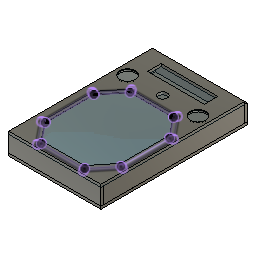
Enclosure Model v2 (Autodesk Fusion 360 design; units mm, degrees)
Autodesk Fusion 360 part; units mm, degrees
sketch "Sketch1" plane through (0, 0, 0) normal (0, 0, 1) x (1, 0, 0) in component "Back"
  line L0 (107.95, 171.45) -> (-107.95, 171.45)
  line L1 (-107.95, 171.45) -> (-107.95, -171.45)
  line L2 (-107.95, -171.45) -> (107.95, -171.45)
  line L3 (107.95, -171.45) -> (107.95, 171.45)
  line L4 (107.95, 171.45) -> (-107.95, -171.45) construction
  line L5 (-107.95, 171.45) -> (107.95, -171.45) construction
  dimension "d1" = 215.9
  dimension "d2" = 342.9
  constraint horizontal L0
  constraint perpendicular L0 L1
  constraint parallel L0 L2
  constraint parallel L1 L3
  constraint coincident L4 origin
  constraint coincident L5 origin
  measures "d1" distance of L1.end L2.end
  measures "d2" distance of L0.end L1.end
extrude "Extrude1" add sketch "Sketch1" along normal blind 6.35 makes body 1 in component "Back"
ref_plane "WorkPlane1" through (0, 131.445, 0) normal (0, 1, 0) x (0, 0, 1) in component "Top/Bottom"
sketch "Sketch1 (2)" plane through (0, 131.445, 0) normal (0, 1, 0) x (1, 0, 0) in component "Top/Bottom"
  line L0 (-101.6, 0) -> (102.87, 0)
  line L1 (102.87, 0) -> (102.87, -50.8)
  line L2 (102.87, -50.8) -> (-101.6, -50.8)
  line L3 (-101.6, -50.8) -> (-101.6, 0)
  dimension "d36" = 204.47
  dimension "d37" = 50.8
  constraint horizontal L0
  constraint vertical L1
  constraint horizontal L2
  constraint vertical L3
  measures "d36" distance of L0.start L0.end
  measures "d37" distance of L0.start L2.end
sketch "Sketch4" plane through (0, 0, 6.35) normal (0, 0, 1) x (-1, 0, 0) in component "Top/Bottom"
  line L0 (-107.95, 171.45) -> (-107.95, -171.45)
  line L1 (-107.95, -171.45) -> (107.95, -171.45)
  line L2 (107.95, -171.45) -> (107.95, 171.45)
  line L3 (107.95, 171.45) -> (-107.95, 171.45)
  line L4 (107.95, -171.45) -> (-107.95, -171.45)
  line L5 (-107.95, -171.45) -> (-107.95, -165.1)
  line L6 (-107.95, -165.1) -> (107.95, -165.1)
  line L7 (107.95, -165.1) -> (107.95, -171.45)
  dimension "d43" = 215.9
  dimension "d44" = 6.35
  constraint horizontal L4
  constraint vertical L5
  constraint horizontal L6
  constraint vertical L7
  constraint coincident L1.end L2.start
  measures "d43" distance of L1.end L0.end
  measures "d44" distance of L1.end L6.end
extrude "Extrude2" add sketch "Sketch4" along normal blind 38.1 separate body contours L0 L1 L2 L4 L5 L6 L7 makes body 2 in component "Top/Bottom"
mirror "Mirror1" about plane through (0, 0, 0) normal (0, 1, 0) of bodies 2 makes body 3 in component "Top/Bottom"
sketch "Sketch1 (3)" plane through (0, 0, 6.35) normal (0, 0, 1) x (-1, 0, 0) in component "Left"
  line L0 (-107.95, 171.45) -> (-107.95, -171.45)
  line L1 (-107.95, -171.45) -> (107.95, -171.45)
  line L2 (107.95, -171.45) -> (107.95, 171.45)
  line L3 (107.95, 171.45) -> (-107.95, 171.45)
  line L4 (107.95, -171.45) -> (107.95, -165.1) construction
  line L5 (107.95, -165.1) -> (101.6, -165.1)
  line L6 (101.6, -165.1) -> (101.6, 165.1)
  line L7 (101.6, 165.1) -> (107.95, 165.1)
  line L8 (107.95, 165.1) -> (107.95, -165.1)
  dimension "d49" = 6.35
  dimension "d50" = 330.2
  constraint coincident L1.end L2.start
  constraint coincident L2 L4.end
  constraint perpendicular L1 L4
  constraint horizontal L5
  constraint vertical L6
  constraint horizontal L7
  constraint vertical L8
  measures "d49" distance of L4.end L5.end
  measures "d50" distance of L4.end L7.end
extrude "Extrude1'" add sketch "Sketch1 (3)" along normal blind 38.1 separate body contours L2 L5 L6 L7 L8 makes body 4 in component "Left"
mirror "Mirror1'" about plane through (0, 0, 0) normal (1, 0, 0) of bodies 4 makes body 5 in component "Left"
sketch "Sketch1 (4)" plane through (0, 0, 44.45) normal (0, 0, 1) x (-1, 0, 0) in component "Lid"
  line L0 (107.95, -165.1) -> (-107.95, -165.1)
  line L1 (-107.95, -165.1) -> (-107.95, -171.45)
  line L2 (-107.95, -171.45) -> (107.95, -171.45)
  line L3 (107.95, -171.45) -> (107.95, -165.1)
  line L4 (107.95, -171.45) -> (-107.95, -171.45)
  line L5 (-107.95, -171.45) -> (-107.95, 171.45)
  line L6 (-107.95, 171.45) -> (107.95, 171.45)
  line L7 (107.95, 171.45) -> (107.95, -171.45)
  dimension "d55" = 215.9
  dimension "d56" = 342.9
  constraint horizontal L4
  constraint vertical L5
  constraint horizontal L6
  constraint vertical L7
  constraint coincident L2.end L3.start
  measures "d55" distance of L2.end L1.end
  measures "d56" distance of L2.end L6.end
extrude "Extrude1''" add sketch "Sketch1 (4)" along normal blind 6.35 separate body contours L0 L5 L6 L7 makes body 6 in component "Lid"
sketch "Sketch2" plane through (0, 0, 50.8) normal (0, 0, 1) x (-1, 0, 0) in component "Lid"
  line L0 (107.95, 171.45) -> (-107.95, 171.45)
  line L1 (-107.95, 171.45) -> (-107.95, -165.1)
  line L2 (-107.95, -165.1) -> (107.95, -165.1)
  line L3 (107.95, -165.1) -> (107.95, 171.45)
  line L4 (0, 171.45) -> (0, 152.4) construction
  line L5 (0, 152.4) -> (0, -50.8) construction
  line L6 (0, -50.8) -> (0, 50.8) construction
  line L7 (0, 50.8) -> (57.15, 50.8) construction
  line L8 (0, 152.4) -> (50.8, 152.4)
  line L9 (50.8, 152.4) -> (50.8, 105.41) construction
  line L10 (50.8, 105.41) -> (88.9, 105.41) construction
  line L11 (50.8, 152.4) -> (88.9, 105.41)
  line L12 (88.9, 105.41) -> (88.9, -8.89)
  line L13 (88.9, -8.89) -> (50.8, -8.89) construction
  line L14 (50.8, -8.89) -> (50.8, -55.88) construction
  line L15 (88.9, -8.89) -> (50.8, -55.88)
  line L16 (50.8, -55.88) -> (0, -55.88)
  line L17 (0, -55.88) -> (0, 152.4)
  dimension "d59" = 19.05
  dimension "d60" = 203.2
  dimension "d61" = 101.6
  dimension "d62" = 57.15
  dimension "d63" = 50.8
  dimension "d64" = 46.99
  dimension "d65" = 38.1
  dimension "d66" = 114.3
  dimension "d67" = 38.1
  dimension "d68" = 46.99
  dimension "d69" = 50.8
  constraint midpoint L0 L4.start
  constraint perpendicular L0 L4
  constraint parallel L4 L5
  constraint parallel L5 L6
  constraint perpendicular L6 L7
  constraint perpendicular L4 L8
  constraint perpendicular L8 L9
  constraint perpendicular L9 L10
  constraint perpendicular L10 L12
  constraint perpendicular L12 L13
  constraint perpendicular L13 L14
  constraint perpendicular L14 L16
  measures "d59" distance of L4.start L4.end
  measures "d60" distance of L4.end L5.end
  measures "d61" distance of L5.end L6.end
  measures "d62" distance of L6.end L7.end
  measures "d63" distance of L4.end L8.end
  measures "d64" distance of L8.end L9.end
  measures "d65" distance of L9.end L10.end
  measures "d66" distance of L10.end L12.end
  measures "d67" distance of L12.end L13.end
  measures "d68" distance of L13.end L14.end
  measures "d69" distance of L14.end L16.end
extrude "Extrude2'" cut sketch "Sketch2" against normal up to surface (6.35 mm away) contours L8 L11 L12 L15 L16 L17 bodies 6 in component "Lid"
mirror "Mirror1''" about plane through (0, 0, 0) normal (1, 0, 0) of "Extrude2'" in component "Lid"
sketch "Sketch3" plane through (0, 0, 50.8) normal (0, 0, 1) x (-1, 0, 0) in component "Lid"
  line L0 (107.95, 171.45) -> (-107.95, 171.45)
  line L1 (-107.95, 171.45) -> (-107.95, -165.1)
  line L2 (-107.95, -165.1) -> (107.95, -165.1)
  line L3 (107.95, -165.1) -> (107.95, 171.45)
  line L4 (50.8, -55.88) -> (-50.8, -55.88)
  line L5 (-50.8, -55.88) -> (-88.9, -8.89)
  line L6 (-88.9, -8.89) -> (-88.9, 105.41)
  line L7 (-88.9, 105.41) -> (-50.8, 152.4)
  line L8 (-50.8, 152.4) -> (50.8, 152.4)
  line L9 (50.8, 152.4) -> (88.9, 105.41)
  line L10 (88.9, 105.41) -> (88.9, -8.89)
  line L11 (88.9, -8.89) -> (50.8, -55.88)
  circle A0 centre (0, -81.28) radius 10.668
  dimension "d74" = 21.336
  dimension "d75" = 25.4
  measures "d74" diameter of A0
  measures "d75" distance of L4 A0.centre
extrude "Extrude3" cut sketch "Sketch3" against normal up to surface (6.35 mm away) contours A0 bodies 6 in component "Lid"
sketch "Sketch4 (2)" plane through (0, 0, 50.8) normal (0, 0, 1) x (-1, 0, 0) in component "Lid"
  circle A0 centre (0, -81.28) radius 10.668
  line L0 (107.95, 171.45) -> (-107.95, 171.45)
  line L1 (-107.95, 171.45) -> (-107.95, -165.1)
  line L2 (-107.95, -165.1) -> (107.95, -165.1)
  line L3 (107.95, -165.1) -> (107.95, 171.45)
  line L4 (50.8, -55.88) -> (-50.8, -55.88)
  line L5 (-50.8, -55.88) -> (-88.9, -8.89)
  line L6 (-88.9, -8.89) -> (-88.9, 105.41)
  line L7 (-88.9, 105.41) -> (-50.8, 152.4)
  line L8 (-50.8, 152.4) -> (50.8, 152.4)
  line L9 (50.8, 152.4) -> (88.9, 105.41)
  line L10 (88.9, 105.41) -> (88.9, -8.89)
  line L11 (88.9, -8.89) -> (50.8, -55.88)
  line L12 (66.675, -144.018) -> (-66.675, -144.018)
  line L13 (-66.675, -144.018) -> (-66.675, -112.268)
  line L14 (-66.675, -112.268) -> (66.675, -112.268)
  line L15 (66.675, -112.268) -> (66.675, -144.018)
  line L16 (66.675, -144.018) -> (-66.675, -112.268) construction
  line L17 (-66.675, -144.018) -> (66.675, -112.268) construction
  point P0 (0, -128.143)
  dimension "d78" = 133.35
  dimension "d79" = 31.75
  dimension "d80" = 30.988
  constraint horizontal L12
  constraint perpendicular L12 L13
  constraint parallel L12 L14
  constraint parallel L13 L15
  constraint coincident L16 P0
  constraint coincident L17 P0
  measures "d78" distance of L13.end L14.end
  measures "d79" distance of L12.end L13.end
  measures "d80" distance of A0.centre L14
extrude "Extrude4" cut sketch "Sketch4 (2)" against normal up to surface (6.35 mm away) contours L12 L13 L14 L15 bodies 6 in component "Lid"
sketch "Sketch5" plane through (0, 0, 44.45) normal (0, 0, -1) x (1, 0, 0) in component "Lid"
  line L0 (-66.675, -144.018) -> (-66.675, -112.268)
  line L1 (-66.675, -112.268) -> (66.675, -112.268)
  line L2 (66.675, -112.268) -> (66.675, -144.018)
  line L3 (66.675, -144.018) -> (-66.675, -144.018)
  circle A0 centre (0, -81.28) radius 10.668
  line L4 (50.8, -55.88) -> (-50.8, -55.88)
  line L5 (-50.8, -55.88) -> (-88.9, -8.89)
  line L6 (-88.9, -8.89) -> (-88.9, 105.41)
  line L7 (-88.9, 105.41) -> (-50.8, 152.4)
  line L8 (-50.8, 152.4) -> (50.8, 152.4)
  line L9 (50.8, 152.4) -> (88.9, 105.41)
  line L10 (88.9, 105.41) -> (88.9, -8.89)
  line L11 (88.9, -8.89) -> (50.8, -55.88)
  line L12 (107.95, 171.45) -> (-107.95, 171.45)
  line L13 (-107.95, 171.45) -> (-107.95, -165.1)
  line L14 (-107.95, -165.1) -> (107.95, -165.1)
  line L15 (107.95, -165.1) -> (107.95, 171.45)
  line L16 (-88.9, -8.89) -> (-50.8, -55.88)
  line L17 (-50.8, -55.88) -> (50.8, -55.88)
  line L18 (-88.9, 105.41) -> (-88.9, -8.89)
  line L19 (50.8, -55.88) -> (88.9, -8.89)
  line L20 (88.9, -8.89) -> (88.9, 105.41)
  line L21 (88.9, 105.41) -> (50.8, 152.4)
  line L22 (-50.8, 152.4) -> (-88.9, 105.41)
  line L23 (50.8, 152.4) -> (-50.8, 152.4)
  line L24 (-50.8, -55.88) -> (50.8, -55.88)
  line L25 (50.8, -55.88) -> (88.9, -8.89)
  line L26 (88.9, 105.41) -> (50.8, 152.4)
  line L27 (50.8, 152.4) -> (-50.8, 152.4)
  line L28 (-50.8, 152.4) -> (-88.9, 105.41)
  line L29 (-88.9, 105.41) -> (-88.9, -8.89)
  line L30 (-88.9, -8.89) -> (-50.8, -55.88)
  constraint coincident L4.end L5.start
  constraint coincident L4.start L11.end
  constraint coincident L10.end L11.start
  constraint coincident L9.end L10.start
  constraint coincident L8.end L9.start
  constraint coincident L7.end L8.start
  constraint coincident L6.end L7.start
  constraint coincident L5.end L6.start
sketch "Sketch1 (5)" plane through (0, 0, 44.45) normal (0, 0, -1) x (1, 0, 0) in component "Punch Box"
  line L0 (-50.8, 152.4) -> (50.8, 152.4)
  line L1 (-88.9, 105.41) -> (-50.8, 152.4)
  line L2 (-88.9, -8.89) -> (-88.9, 105.41)
  line L3 (-50.8, -55.88) -> (-88.9, -8.89)
  line L4 (50.8, -55.88) -> (-50.8, -55.88)
  line L5 (88.9, -8.89) -> (50.8, -55.88)
  line L6 (88.9, 105.41) -> (88.9, -8.89)
  line L7 (50.8, 152.4) -> (88.9, 105.41)
  line L8 (53.8264, 158.75) -> (95.25, 107.6609)
  line L9 (95.25, 107.6609) -> (95.25, -11.1409)
  line L10 (95.25, -11.1409) -> (53.8264, -62.23)
  line L11 (53.8264, -62.23) -> (-53.8264, -62.23)
  line L12 (-53.8264, -62.23) -> (-95.25, -11.1409)
  line L13 (-95.25, -11.1409) -> (-95.25, 107.6609)
  line L14 (-95.25, 107.6609) -> (-53.8264, 158.75)
  line L15 (-53.8264, 158.75) -> (53.8264, 158.75)
  line L16 (98.425, 108.7863) -> (98.425, -12.2663)
  line L17 (98.425, -12.2663) -> (55.3396, -65.405)
  line L18 (55.3396, -65.405) -> (-55.3396, -65.405)
  line L19 (-55.3396, -65.405) -> (-98.425, -12.2663)
  line L20 (-98.425, -12.2663) -> (-98.425, 108.7863)
  line L21 (-98.425, 108.7863) -> (-55.3396, 161.925)
  line L22 (-55.3396, 161.925) -> (55.3396, 161.925)
  line L23 (55.3396, 161.925) -> (98.425, 108.7863)
  dimension "d83" = -6.35
  dimension "d84" = -9.525
extrude "Extrude1'''" add sketch "Sketch1 (5)" along normal blind 34.925 separate body contours L16 L17 L18 L19 L20 L21 L22 L23 makes body 7 in component "Punch Box"
sketch "Sketch5 (2)" plane through (0, 0, 9.525) normal (0, 0, -1) x (1, 0, 0) in component "Punch Box"
  line L0 (-95.25, 107.6609) -> (-53.8264, 158.75)
  line L1 (-53.8264, 158.75) -> (53.8264, 158.75)
  line L2 (53.8264, 158.75) -> (95.25, 107.6609)
  line L3 (95.25, 107.6609) -> (95.25, -11.1409)
  line L4 (95.25, -11.1409) -> (53.8264, -62.23)
  line L5 (53.8264, -62.23) -> (-53.8264, -62.23)
  line L6 (-53.8264, -62.23) -> (-95.25, -11.1409)
  line L7 (-95.25, -11.1409) -> (-95.25, 107.6609)
  line L8 (55.3396, 161.925) -> (-55.3396, 161.925)
  line L9 (-55.3396, 161.925) -> (-98.425, 108.7863)
  line L10 (-98.425, 108.7863) -> (-98.425, -12.2663)
  line L11 (-98.425, -12.2663) -> (-55.3396, -65.405)
  line L12 (-55.3396, -65.405) -> (55.3396, -65.405)
  line L13 (55.3396, -65.405) -> (98.425, -12.2663)
  line L14 (98.425, -12.2663) -> (98.425, 108.7863)
  line L15 (98.425, 108.7863) -> (55.3396, 161.925)
  line L16 (55.3396, -65.405) -> (-55.3396, -65.405)
  line L17 (-55.3396, -65.405) -> (-98.425, -12.2663)
  line L18 (-98.425, 108.7863) -> (-98.425, -12.2663)
  line L19 (-98.425, 108.7863) -> (-55.3396, 161.925)
  line L20 (-55.3396, 161.925) -> (55.3396, 161.925)
  line L21 (98.425, 108.7863) -> (55.3396, 161.925)
  line L22 (98.425, 108.7863) -> (98.425, -12.2663)
  line L23 (98.425, -12.2663) -> (55.3396, -65.405)
  constraint coincident L12.end L13.start
  constraint coincident L11.end L12.start
  constraint coincident L10.end L11.start
  constraint coincident L9.end L10.start
  constraint coincident L8.end L9.start
  constraint coincident L8.start L15.end
  constraint coincident L14.end L15.start
  constraint parallel L15 L21
  constraint coincident L13.end L14.start
extrude "Extrude2''" add sketch "Sketch5 (2)" along normal blind 3.175 separate body contours L0 L1 L2 L3 L4 L5 L6 L7 makes body 8 in component "Punch Box"
sketch "Sketch1 (6)" plane through (0, 0, 44.45) normal (0, 0, -1) x (1, 0, 0) in component "Punch Pad"
  line L0 (53.8264, -62.23) -> (-53.8264, -62.23)
  line L1 (-53.8264, -62.23) -> (-95.25, -11.1409)
  line L2 (-95.25, -11.1409) -> (-95.25, 107.6609)
  line L3 (95.25, -11.1409) -> (53.8264, -62.23)
  line L4 (95.25, 107.6609) -> (95.25, -11.1409)
  line L5 (53.8264, 158.75) -> (95.25, 107.6609)
  line L6 (-53.8264, 158.75) -> (53.8264, 158.75)
  line L7 (-95.25, 107.6609) -> (-53.8264, 158.75)
extrude "Extrude1''''" add sketch "Sketch1 (5)" along normal blind 3.175 separate body contours L0 L1 L2 L3 L4 L5 L6 L7 makes body 9 in component "Punch Pad"
sketch "Sketch8" plane through (0, 0, 44.45) normal (0, 0, -1) x (1, 0, 0) in component "Lid"
  line L0 (107.8877, -81.5117) -> (82.4877, -81.5117) construction
  circle A0 centre (82.4877, -81.5117) radius 18.161
  dimension "d91" = 25.4
  dimension "d92" = 36.322
  constraint coincident L0.end A0.centre
  measures "d91" distance of L0.start L0.end
  measures "d92" diameter of A0
extrude "Extrude5" cut sketch "Sketch8" against normal up to surface (6.35 mm away) bodies 6 in component "Lid"
sketch "Sketch9" plane through (0, 0, 44.45) normal (0, 0, -1) x (1, 0, 0) in component "Lid"
  circle A0 centre (82.4879, -81.5112) radius 19.812
  dimension "d95" = 39.624
  measures "d95" diameter of A0
extrude "Extrude6" cut sketch "Sketch9" against normal up to surface (4.572 mm away) bodies 6 in component "Lid"
mirror "Mirror2" about plane through (0, 0, 0) normal (1, 0, 0) of "Extrude5", "Extrude6" in component "Lid"
component "Back" placed x (1, 0, 0) y (0, 1, 0) z (0, 0, 1) at (0, 0, 0)
component "Top/Bottom" placed x (1, 0, 0) y (0, 1, 0) z (0, 0, 1) at (0, 0, 0)
component "Left" placed x (1, 0, 0) y (0, 1, 0) z (0, 0, 1) at (0, 0, 0)
component "Right" placed x (1, 0, 0) y (0, 1, 0) z (0, 0, 1) at (0, 0, 0)
component "Lid" placed x (1, 0, 0) y (0, 1, 0) z (0, 0, 1) at (0, 0, 0)
component "Punch Box" placed x (1, 0, 0) y (0, 1, 0) z (0, 0, 1) at (0, 0, 0)
component "Punch Pad" placed x (1, 0, 0) y (0, 1, 0) z (0, 0, 1) at (0, 0, 0)
equation "d3 = ( 1 / 4 ) * 1 in"
equation "d85 = 1.50 in - ( 1 / 8 ) * 1 in"
equation "d87 = ( 1 / 8 ) * 1 in"
equation "d89 = ( 1 / 8 ) * 1 in"
